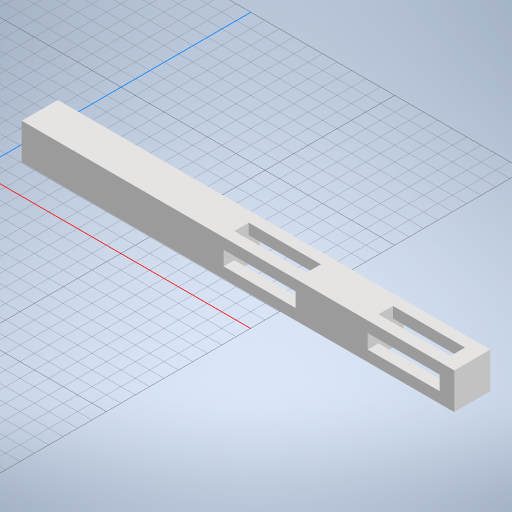
# Autodesk Inventor part: 1_inner_leg
Saved by Autodesk Inventor 2024 (Build 280153000, 153)
## iProperties
Created: 2023-05-22
Part Number: 1_inner_leg
Material: Generic
Document SubType Name: Modeling
Designer: aasmu
Density: 1 g/cm^3
Appearance: Default
Author: aasmu
Autodesk Inventor part; units mm, degrees
ref_plane "YZ Plane" through (0, 0, 0) normal (1, 0, 0) x (0, 1, 0)
ref_plane "XZ Plane" through (0, 0, 0) normal (0, 1, 0) x (-1, 0, 0)
ref_plane "XY Plane" through (0, 0, 0) normal (0, 0, 1) x (1, 0, 0)
sketch "Sketch1" plane through (0, 0, 0) normal (0, 1, 0) x (-1, 0, 0)
  line L0 (-21.8006, -40.7032) -> (-621.8006, -40.7032)
  line L1 (-621.8006, -40.7032) -> (-621.8006, -90.7032)
  line L2 (-621.8006, -90.7032) -> (-21.8006, -90.7032)
  line L3 (-21.8006, -90.7032) -> (-21.8006, -40.7032)
  line L4 (-301.8006, -75.7032) -> (-301.8006, -55.7032)
  line L5 (-601.8006, -55.7032) -> (-601.8006, -75.7032)
  line L6 (-601.8006, -75.7032) -> (-501.8006, -75.7032)
  line L7 (-501.8006, -75.7032) -> (-501.8006, -55.7032)
  line L8 (-501.8006, -55.7032) -> (-601.8006, -55.7032)
  line L9 (-301.8006, -75.7032) -> (-401.8006, -75.7032)
  line L10 (-401.8006, -75.7032) -> (-401.8006, -55.7032)
  line L11 (-401.8006, -55.7032) -> (-301.8006, -55.7032)
  line L12 (-401.8006, -75.7032) -> (-501.8006, -75.7032)
  line L13 (-401.8006, -55.7032) -> (-501.8006, -55.7032)
  line L14 (-601.8006, -65.7032) -> (-621.8006, -65.7032)
  point P0 (0, 0)
  dimension "leg_length" = 600
  dimension "leg_witdh" = 50
  dimension "rail_length" = 300
  dimension "rail_depth" = 20
  dimension "d5" = 100
  dimension "d6" = 20
  constraints: 30 end point, 5 perpendicular, 4 horizontal, 4 vertical, 2 equal length, 2 midpoint, 2 point on line, 1 collinear, 1 other
  measures "leg_length" distance of L0.start L0.end
  measures "leg_witdh" distance of L2.end L0.start
  measures "rail_length" distance of L5.end L4.start
  measures "rail_depth" distance from line of L1 L5.end
  measures "d5" distance of L9.end L6.end
  measures "d6" distance of L5.start L5.end
extrude "Extrusion1" add sketch "Sketch1" along normal blind 50 contours L3 L2 L1 L0 | L12 L7 L13 L10
sketch "Sketch2" plane through (21.8006, 0, -40.7032) normal (0, 0, 1) x (1, 0, 0)
  line L0 (580, 0) -> (580, 50) projected
  line L1 (280, 0) -> (280, 50) projected
  line L2 (380, 0) -> (380, 50) projected
  line L3 (280, 35) -> (380, 35)
  line L4 (380, 35) -> (380, 15)
  line L5 (380, 15) -> (280, 15)
  line L6 (280, 15) -> (280, 35)
  line L7 (480, 0) -> (480, 50) projected
  line L8 (580, 35) -> (480, 35)
  line L9 (480, 35) -> (480, 15)
  line L10 (480, 15) -> (580, 15)
  line L11 (580, 15) -> (580, 35)
  line L12 (328.2754, 15) -> (328.2754, 0)
  line L13 (600, 0) -> (0, 0) projected
  line L14 (328.2754, 35) -> (328.2754, 50)
  line L15 (0, 50) -> (600, 50) projected
  point P0 (-21.8006, 0)
  point P1 (380, 25)
  dimension "d11" = 20
  constraints: 20 end point, 10 point on line, 4 parallel, 3 collinear, 2 horizontal, 2 perpendicular, 1 midpoint, 1 vertical
  measures "d11" distance of L3.end L4.end
extrude "Extrusion2" cut sketch "Sketch2" against normal blind 50 contours L10 L7 L8 L0 | L5 L1 L3 L2
equation "\"rail_length\" = 0.5 * leg_length"
equation "\"d11\" = rail_depth"
equation "\"d12\" = d7"
equation "\"d7\" = 50"
body "Solid1"
